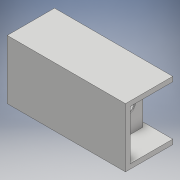
# Autodesk Inventor part: BoxBase
Saved by Autodesk Inventor 2018 (Build 220112000, 112)
## iProperties
Created: 2019-07-19
Part Number: BoxBase
Material: Generic
Document SubType Name: Modeling
Designer: aal_9
Density: 1 g/cm^3
Appearance: Default
Author: aal_9
Autodesk Inventor part; units mm, degrees
ref_plane "YZ Plane" through (0, 0, 0) normal (1, 0, 0) x (0, 1, 0)
ref_plane "XZ Plane" through (0, 0, 0) normal (0, 1, 0) x (-1, 0, 0)
ref_plane "XY Plane" through (0, 0, 0) normal (0, 0, 1) x (1, 0, 0)
sketch "Sketch1" plane through (0, 0, 0) normal (0, 1, 0) x (-1, 0, 0)
  line L0 (50, -25) -> (-50, -25)
  line L1 (-50, -25) -> (-50, 25)
  line L2 (-50, 25) -> (50, 25)
  line L3 (50, 25) -> (50, -25)
  point P0 (0, 0)
  dimension "d0" = 100
  dimension "d1" = 50
  dimension "d2" = 25
  dimension "d3" = 50
  constraints: 8 end point, 2 parallel, 1 horizontal, 1 perpendicular
  measures "d0" distance of L1.end L2.end
  measures "d1" distance of L0.end L1.end
  measures "d2" distance from line of point (0, 0) L0
  measures "d3" distance from line of point (0, 0) L3
extrude "Extrusion1" add sketch "Sketch1" along normal blind 4
sketch "Sketch2" plane through (0, 4, 0) normal (0, 1, 0) x (1, 0, 0)
  line L0 (50, -25) -> (-50, -25)
  line L1 (-50, -25) -> (-50, -21)
  line L2 (-50, -21) -> (50, -21)
  line L3 (50, -21) -> (50, -25)
  line L4 (50, 25) -> (-50, 25)
  line L5 (-50, 25) -> (-50, 21)
  line L6 (-50, 21) -> (50, 21)
  line L7 (50, 21) -> (50, 25)
  point P0 (0, 0)
  dimension "d7" = 100
  dimension "d8" = 4
  dimension "d10" = 4
  constraints: 16 end point, 4 parallel, 2 horizontal, 2 perpendicular, 1 point on line
  measures "d7" distance of L1.end L2.end
  measures "d8" distance of L0.end L1.end
  measures "d10" distance of L5.end L4.end
extrude "Extrusion2" add sketch "Sketch2" along normal blind 36
sketch "Sketch3" plane through (0, 4, 0) normal (0, 1, 0) x (1, 0, 0)
  line L0 (50, 21) -> (-50, 21) projected
  line L1 (28.6, 21) -> (25.6, 21)
  line L2 (25.6, 21) -> (25.6, -21)
  line L3 (25.6, -21) -> (28.6, -21)
  line L4 (28.6, -21) -> (28.6, 21)
  line L5 (50, -21) -> (50, 21) projected
  line L6 (50, -21) -> (-50, -21) projected
  point P0 (0, 0)
  dimension "d15" = 21.4
  dimension "d16" = 0
  dimension "d17" = 3
  constraints: 8 end point, 2 parallel, 1 horizontal, 1 perpendicular, 1 point on line
  measures "d15" distance between parallel lines of L5 L4
  measures "d16" distance between parallel lines of L6 L3
  measures "d17" distance between parallel lines of L4 L2
extrude "Extrusion3" add sketch "Sketch3" along normal blind 32 contours L4 L3 L2 L0
sketch "Sketch4" plane through (28.6, 4, 21) normal (1, 0, 0) x (0, 0, -1)
  circle A0 centre (21, 20) radius 5
  line L0 (0, 0) -> (42, 0) projected
  line L1 (0, 0) -> (0, 36) projected
  circle A1 centre (13.6, 20) radius 1.25
  point P0 (21, -4)
  dimension "d20" = 10
  dimension "d22" = 21
  dimension "d23" = 2.5
  dimension "d24" = 7.4
  dimension "d28" = 20
  dimension "d29" = 20
  constraints: 2 centre point
  measures "d20" diameter of A0
  measures "d22" distance from line of L1 A0.centre
  measures "d23" diameter of A1
  measures "d24" distance of A0.centre A1.centre
  measures "d28" distance from line of L0 A0.centre
  measures "d29" distance from line of L0 A1.centre
extrude "Extrusion4" cut sketch "Sketch4" against normal up to next
sketch "Sketch5" plane through (28.6, 4, 21) normal (1, 0, 0) x (0, 0, -1)
  circle A0 centre (21, 20) radius 5 projected
  circle A1 centre (21, 20) radius 5.85
  point P0 (21, -4)
  dimension "d30" = 11.7
  constraints: 1 centre point, 1 coincident
  measures "d30" diameter of A1
extrude "Extrusion5" cut sketch "Sketch5" against normal blind 0.5
sketch "Sketch6" plane through (0, 4, 0) normal (0, 1, 0) x (1, 0, 0)
  line L0 (8.6, -21) -> (5.6, -21)
  line L1 (5.6, -21) -> (5.6, 21.1393)
  line L2 (5.6, 21.1393) -> (8.6, 21.1393)
  line L3 (8.6, 21.1393) -> (8.6, -21)
  line L4 (25.6, -21) -> (25.6, 21) projected
  line L5 (50, -21) -> (-50, -21) projected
  line L6 (-50, 21) -> (-50, -21) projected
  point P0 (0, 0)
  dimension "d34" = 3
  dimension "d35" = 0
  dimension "d52" = 55.6
  constraints: 8 end point, 2 parallel, 1 horizontal, 1 perpendicular
  measures "d34" distance between parallel lines of L1 L3
  measures "d35" distance between parallel lines of L5 L0
  measures "d52" distance between parallel lines of L6 L1
extrude "Extrusion6" add sketch "Sketch6" along normal blind 20
sketch "Sketch7" plane through (5.6, 4, -21) normal (-1, 0, 0) x (0, 0, 1)
  circle A0 centre (21, 20) radius 5 projected
  circle A1 centre (21, 20) radius 5
  point P0 (21, -4)
  dimension "d38" = 10
  constraints: 1 centre point, 1 coincident
  measures "d38" diameter of A1
extrude "Extrusion7" cut sketch "Sketch7" against normal up to next
sketch "Sketch8" plane through (5.6, 4, -21) normal (-1, 0, 0) x (0, 0, 1)
  line L0 (8, 13) -> (17, 13)
  line L1 (17, 13) -> (17, 10)
  line L2 (17, 10) -> (8, 10)
  line L3 (8, 10) -> (8, 13)
  line L4 (0, 0) -> (0, 36) projected
  line L5 (0, 0) -> (42, 0) projected
  point P0 (21, -4)
  dimension "d41" = 8
  dimension "d42" = 9
  dimension "d43" = 10
  dimension "d44" = 3
  constraints: 8 end point, 2 parallel, 1 horizontal, 1 perpendicular
  measures "d41" distance between parallel lines of L4 L3
  measures "d42" distance of L0.start L0.end
  measures "d43" distance between parallel lines of L5 L2
  measures "d44" distance of L0.end L1.end
extrude "Extrusion8" add sketch "Sketch8" along normal blind 6.1
sketch "Sketch10" plane through (0, 4, 0) normal (0, 1, 0) x (1, 0, 0)
  line L0 (-50, -21) -> (-50, -25) projected
  line L1 (-50, 21) -> (50, 21) projected
  line L2 (-50, -21) -> (-46, -21)
  line L3 (-46, -21) -> (-46, 21)
  line L4 (-46, 21) -> (-50, 21)
  line L5 (-50, 21) -> (-50, -21)
  point P0 (0, 0)
  dimension "d53" = 4
  constraints: 8 end point, 2 parallel, 1 horizontal, 1 perpendicular, 1 point on line
  measures "d53" distance of L0.start L2.end
extrude "Extrusion10" add sketch "Sketch10" along normal blind 20
sketch "Sketch11" plane through (-50, 0, -25) normal (-1, 0, 0) x (0, 0, 1)
  circle A0 centre (25, 24) radius 7.5
  point P0 (25, 0)
  dimension "d56" = 15
  constraints: 1 centre point, 1 coincident
  measures "d56" diameter of A0
extrude "Extrusion11" cut sketch "Sketch11" against normal up to surface (4 mm away)
sketch "Sketch12" plane through (-46, 4, 21) normal (1, 0, 0) x (0, 0, -1)
  line L0 (34, 13) -> (25, 13)
  line L1 (25, 13) -> (25, 10)
  line L2 (25, 10) -> (34, 10)
  line L3 (34, 10) -> (34, 13)
  line L4 (42, 20) -> (42, 36) projected
  line L5 (-4, -4) -> (46, -4) projected
  point P0 (21, -4)
  dimension "d59" = 9
  dimension "d60" = 8
  dimension "d61" = 3
  dimension "d62" = 14
  constraints: 8 end point, 2 parallel, 1 horizontal, 1 perpendicular
  measures "d59" distance of L0.start L0.end
  measures "d60" distance between parallel lines of L4 L3
  measures "d61" distance between parallel lines of L2 L0
  measures "d62" distance between parallel lines of L5 L2
extrude "Extrusion12" add sketch "Sketch12" along normal blind 8.5
sketch "Sketch9" plane through (5.6, 17, -4) normal (0, 1, 0) x (1, 0, 0)
  line L0 (0, 17) -> (0, 1) projected
  line L1 (-51.6, 3.5) -> (-51.6, 17) projected
  line L2 (-51.6, 9) -> (-43.1, 9) projected
  line L3 (-45.1, 5.5) -> (-45.1, 3.5) construction
  line L4 (-46.1, 5.5) -> (-46.1, 3.5)
  line L5 (-44.1, 3.5) -> (-44.1, 5.5)
  arc A0 (-44.1, 5.5) -> (-46.1, 5.5) centre (-45.1, 5.5) ccw
  arc A1 (-46.1, 3.5) -> (-44.1, 3.5) centre (-45.1, 3.5) ccw
  line L6 (-4.1, 5.5) -> (-4.1, 3.5) construction
  line L7 (-5.1, 5.5) -> (-5.1, 3.5)
  line L8 (-3.1, 3.5) -> (-3.1, 5.5)
  arc A2 (-3.1, 5.5) -> (-5.1, 5.5) centre (-4.1, 5.5) ccw
  arc A3 (-5.1, 3.5) -> (-3.1, 3.5) centre (-4.1, 3.5) ccw
  line L9 (0, 9) -> (-6.1, 9) projected
  point P0 (-5.6, -4)
  point P1 (-45.1, 4.5)
  point P2 (-4.1, 4.5)
  dimension "d68" = 2
  dimension "d70" = 2
  dimension "d71" = 6.5
  dimension "d72" = 2
  dimension "d73" = 2
  dimension "d74" = 4.1
  dimension "d75" = 4.5
  dimension "d76" = 4.5
  constraints: 16 end point, 8 point on circle, 8 tangent, 4 centre point, 2 midpoint, 2 parallel, 2 vertical
  measures "d68" distance of L3.end L3.start
  measures "d70" distance between parallel lines of L4 L5
  measures "d71" distance from line of L1 point (-45.1, 4.5)
  measures "d72" distance of L6.start L6.end
  measures "d73" diameter of A3
  measures "d74" distance from line of L0 point (-4.1, 4.5)
  measures "d75" distance from line of L9 point (-4.1, 4.5)
  measures "d76" distance from line of L2 point (-45.1, 4.5)
extrude "Extrusion9" cut sketch "Sketch9" against normal blind 3
sketch "Sketch13" plane through (0, 40, 0) normal (0, 1, 0) x (1, 0, 0)
  line L0 (-48, 21) -> (-46, 21)
  line L1 (-46, 21) -> (-46, 23)
  line L2 (-46, 23) -> (-48, 23)
  line L3 (-48, 23) -> (-48, 21)
  line L4 (-50, 21) -> (50, 21) projected
  line L5 (-50, 25) -> (-50, 21) projected
  line L6 (-48, -23) -> (-46, -23)
  line L7 (-46, -23) -> (-46, -21)
  line L8 (-46, -21) -> (-48, -21)
  line L9 (-48, -21) -> (-48, -23)
  line L10 (-50, -21) -> (-50, -25) projected
  line L11 (50, -21) -> (-50, -21) projected
  point P0 (0, 0)
  dimension "d77" = 2
  dimension "d78" = 2
  dimension "d79" = 0
  dimension "d80" = 2
  dimension "d81" = 2
  dimension "d82" = 2
  dimension "d83" = 2
  dimension "d84" = 0
  constraints: 16 end point, 4 parallel, 2 horizontal, 2 perpendicular
  measures "d77" distance of L2.end L1.end
  measures "d78" distance of L1.end L0.end
  measures "d79" distance between parallel lines of L4 L0
  measures "d80" distance between parallel lines of L5 L3
  measures "d81" distance of L8.end L7.end
  measures "d82" distance of L7.end L6.end
  measures "d83" distance between parallel lines of L10 L9
  measures "d84" distance between parallel lines of L11 L8
extrude "Extrusion13" cut sketch "Sketch13" against normal up to surface (16 mm away)
sketch "Sketch14" plane through (28.6, 4, 21) normal (1, 0, 0) x (0, 0, -1)
  line L0 (0, 0) -> (42, 0) projected
  line L1 (42, 0) -> (32, 0)
  line L2 (32, 0) -> (32, 5)
  line L3 (32, 5) -> (42, 5)
  line L4 (42, 5) -> (42, 0)
  point P0 (21, -4)
  dimension "d87" = 10
  dimension "d88" = 5
  constraints: 8 end point, 2 parallel, 1 horizontal, 1 perpendicular
  measures "d87" distance of L2.end L3.end
  measures "d88" distance of L1.end L2.end
extrude "Extrusion14" cut sketch "Sketch14" against normal up to surface (23 mm away)
body "Solid1"
